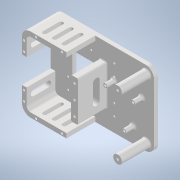
# Autodesk Inventor part: fleet
Saved by Autodesk Inventor 2020 (Build 240168000, 168)
## iProperties
Created: 2020-01-06
Part Number: fleet
Material: Generic
Document SubType Name: Modeling
Designer: my
Density: 1 g/cm^3
Appearance: Default
Author: my
Autodesk Inventor part; units mm, degrees
ref_plane "YZ Plane" through (0, 0, 0) normal (1, 0, 0) x (0, 1, 0)
ref_plane "XZ Plane" through (0, 0, 0) normal (0, 1, 0) x (-1, 0, 0)
ref_plane "XY Plane" through (0, 0, 0) normal (0, 0, 1) x (1, 0, 0)
sketch "Sketch1" plane through (0, 0, 0) normal (0, 0, 1) x (1, 0, 0)
  line L0 (-75, -65) -> (75, -65)
  line L1 (90, -50) -> (90, 50)
  line L2 (75, 65) -> (-75, 65)
  line L3 (-90, 50) -> (-90, -50)
  line L4 (-90, -65) -> (90, 65) construction
  line L5 (90, -65) -> (-90, 65) construction
  arc A0 (75, -65) -> (90, -50) centre (75, -50) ccw
  arc A1 (90, 50) -> (75, 65) centre (75, 50) ccw
  arc A2 (-75, 65) -> (-90, 50) centre (-75, 50) ccw
  arc A3 (-90, -50) -> (-75, -65) centre (-75, -50) ccw
  point P0 (0, 0)
  dimension "d0" = 180
  dimension "d1" = 130
  dimension "d9" = 15
  dimension "d10" = 15
  constraints: 12 end point, 8 point on circle, 8 point on line, 8 tangent, 4 centre point, 2 equal radius, 2 midpoint, 2 parallel, 1 horizontal, 1 perpendicular
  measures "d0" distance of L4.end L5.end
  measures "d1" distance of L5.start L4.end
  measures "d9" radius of A0
  measures "d10" radius of A1
extrude "Extrusion1" add sketch "Sketch1" along normal blind 7
sketch "Sketch3" plane through (0, 0, 7) normal (0, 0, 1) x (1, 0, 0)
  circle A0 centre (76.5, -52) radius 7.5
  circle A1 centre (76.5, 52) radius 7.5
  line L0 (7.5, 30) -> (-4.5, 30)
  line L1 (-4.5, 30) -> (-4.5, -30)
  line L2 (-4.5, -30) -> (7.5, -30)
  line L3 (7.5, -30) -> (7.5, 30)
  line L4 (7.5, 30) -> (-4.5, -30) construction
  line L5 (-4.5, 30) -> (7.5, -30) construction
  point P0 (1.5, 0)
  point P1 (0, 0)
  dimension "d11" = 15
  dimension "d12" = 104
  dimension "d13" = 52
  dimension "d14" = 75
  dimension "d15" = 12
  dimension "d16" = 60
  dimension "d17" = 7.5
  dimension "d18" = 30
  constraints: 12 end point, 2 centre point, 2 midpoint, 2 parallel, 1 equal radius, 1 horizontal, 1 perpendicular, 1 vertical alignment
  measures "d11" diameter of A0
  measures "d12" distance of A1.centre A0.centre
  measures "d13" vertical distance of point (1.5, 0) A0.centre
  measures "d14" horizontal distance of A0.centre point (1.5, 0)
  measures "d15" distance of L1.end L2.end
  measures "d16" distance of L0.end L1.end
  measures "d17" distance from line of point (0, 0) L3
  measures "d18" distance from line of L2 point (0, 0)
extrude "Extrusion2" add sketch "Sketch3" along normal blind 50
sketch "Sketch4" plane through (0, 0, 7) normal (0, 0, 1) x (1, 0, 0)
  line L0 (-12.5, 23) -> (-52.5, 23)
  line L1 (-52.5, 23) -> (-52.5, -23)
  line L2 (-52.5, -23) -> (-12.5, -23)
  line L3 (-12.5, -23) -> (-12.5, 23)
  line L4 (-12.5, 23) -> (-52.5, -23) construction
  line L5 (-52.5, 23) -> (-12.5, -23) construction
  line L6 (-4.5, -30) -> (-4.5, 30) projected
  point P0 (0, 0)
  point P1 (-32.5, 0)
  dimension "d21" = 46
  dimension "d22" = 40
  dimension "d25" = 28
  constraints: 12 end point, 2 midpoint, 2 parallel, 1 horizontal, 1 horizontal alignment, 1 perpendicular
  measures "d21" distance of L2.end L0.start
  measures "d22" distance of L1.end L2.end
  measures "d25" distance from line of L6 point (-32.5, 0)
extrude "Extrusion3" cut sketch "Sketch4" against normal mid plane 50
fillet "Fillet1" radius 2 8 edges at (1.5, 30, 7) (7.5, 0, 7) (7.5, 30, 32) (-4.5, 30, 32) (-4.5, 0, 7) (-4.5, -30, 32) (1.5, -30, 7) (7.5, -30, 32)
sketch "Sketch5" plane through (0, 0, 7) normal (0, 0, 1) x (1, 0, 0)
  arc A0 (90, 50) -> (75, 65) centre (75, 50) ccw projected
  line L0 (75, 65) -> (-75, 65) projected
  arc A1 (-75, 65) -> (-90, 50) centre (-75, 50) ccw projected
  line L1 (-90, 50) -> (-90, -50) projected
  arc A2 (-90, -50) -> (-75, -65) centre (-75, -50) ccw projected
  line L2 (-75, -65) -> (75, -65) projected
  arc A3 (75, -65) -> (90, -50) centre (75, -50) ccw projected
  line L3 (90, -50) -> (90, 50) projected
  circle A4 centre (76.5, -52) radius 7.5 projected
  circle A5 centre (76.5, 52) radius 7.5 projected
  line L4 (-52.5, 23) -> (-12.5, 23) projected
  line L5 (-12.5, 23) -> (-12.5, -23) projected
  line L6 (-12.5, -23) -> (-52.5, -23) projected
  line L7 (-52.5, -23) -> (-52.5, 23) projected
  arc A6 (-2.5, 32) -> (-6.5, 28) centre (-2.5, 28) ccw projected
  line L8 (5.5, 32) -> (-2.5, 32) projected
  arc A7 (9.5, 28) -> (5.5, 32) centre (5.5, 28) ccw projected
  line L9 (9.5, -28) -> (9.5, 28) projected
  arc A8 (5.5, -32) -> (9.5, -28) centre (5.5, -28) ccw projected
  line L10 (-2.5, -32) -> (5.5, -32) projected
  arc A9 (-6.5, -28) -> (-2.5, -32) centre (-2.5, -28) ccw projected
  line L11 (-6.5, 28) -> (-6.5, -28) projected
  line L12 (75, -57) -> (-75, -57)
  arc A10 (-82, -50) -> (-75, -57) centre (-75, -50) ccw
  line L13 (-82, -50) -> (-82, 50)
  arc A11 (-75, 57) -> (-82, 50) centre (-75, 50) ccw
  line L14 (-75, 57) -> (75, 57)
  arc A12 (82, 50) -> (75, 57) centre (75, 50) ccw
  line L15 (82, 50) -> (82, -50)
  arc A13 (75, -57) -> (82, -50) centre (75, -50) ccw
  line L16 (-82, -23) -> (-90, -23)
  line L17 (-82, 23) -> (-90, 23)
  line L18 (-12.5, -57) -> (-12.5, -65)
  line L19 (-12.5, 57) -> (-12.5, 65)
  line L20 (75, 65) -> (-75, 65) projected
  point P0 (0, 0)
  dimension "d27" = 8
  constraints: 16 end point, 14 point on line, 8 point on circle, 4 centre point, 1 collinear, 1 perpendicular, 7 other
  measures "d27" distance between parallel lines of L12 L2
extrude "Extrusion4" add sketch "Sketch5" along normal blind 50 contours L19 L14 A11 L13 L17 L1 A1 L0 | L2 A2 L1 L16 L13 A10 L12 L18
sketch "Sketch6" plane through (76.5, -52, 57) normal (0, 0, 1) x (1, 0, 0)
  circle A0 centre (0, 0) radius 7.5 projected
  circle A1 centre (0, 0) radius 2
  circle A2 centre (0, 104) radius 7.5 projected
  circle A3 centre (0, 104) radius 2
  circle A4 centre (-75, 27) radius 2
  circle A5 centre (-75, 52) radius 2
  circle A6 centre (-75, 77) radius 2
  circle A7 centre (-97, -9.5) radius 2
  circle A8 centre (-142, -9.5) radius 2
  circle A9 centre (-163, 6) radius 2
  circle A10 centre (-163, 23) radius 2
  circle A11 centre (-163, 81) radius 2
  circle A12 centre (-163, 98) radius 2
  circle A13 centre (-142, 113.5) radius 2
  circle A14 centre (-97, 113.5) radius 2
  line L0 (-81, 80) -> (-81, 24) projected
  line L1 (-151.5, -13) -> (-89, -13) projected
  line L2 (-89, -13) -> (-89, -5) projected
  line L3 (-166.5, 29) -> (-166.5, 2) projected
  line L4 (-158.5, 29) -> (-166.5, 29) projected
  line L5 (-166.5, 75) -> (-158.5, 75) projected
  line L6 (-166.5, 102) -> (-166.5, 75) projected
  line L7 (-89, 117) -> (-151.5, 117) projected
  point P0 (-76.5, 52)
  dimension "d30" = 4
  dimension "d31" = 6
  dimension "d32" = 25
  dimension "d33" = 25
  dimension "d34" = 45
  dimension "d35" = 3.5
  dimension "d36" = 8
  dimension "d37" = 3.5
  dimension "d38" = 17
  dimension "d39" = 6
  dimension "d40" = 6
  dimension "d41" = 3.5
  dimension "d42" = 17
  dimension "d43" = 3.5
  constraints: 13 centre point, 12 equal radius, 6 vertical alignment, 3 horizontal alignment, 2 coincident
  measures "d30" diameter of A1
  measures "d31" distance from line of A4.centre L0
  measures "d32" distance of A5.centre A4.centre
  measures "d33" distance of A6.centre A5.centre
  measures "d34" distance of A8.centre A7.centre
  measures "d35" distance from line of L1 A7.centre
  measures "d36" distance from line of A7.centre L2
  measures "d37" distance from line of L3 A9.centre
  measures "d38" distance of A10.centre A9.centre
  measures "d39" distance from line of L4 A10.centre
  measures "d40" distance from line of A11.centre L5
  measures "d41" distance from line of L6 A11.centre
  measures "d42" distance of A12.centre A11.centre
  measures "d43" distance from line of A14.centre L7
extrude "Extrusion5" cut sketch "Sketch6" against normal blind 10 contours A1 | A3 | A4 | A5 | A6 | A7 | A8 | A9 | A10 | A11 | A12 | A13 | A14
sketch "Sketch7" plane through (0, 0, 7) normal (0, 0, 1) x (1, 0, 0)
  point P0 (0, 0)
sketch "Sketch8" plane through (0, 0, 7) normal (0, 0, 1) x (1, 0, 0)
  circle A0 centre (20.7748, 40) radius 1.7 projected
  circle A1 centre (-59.5, 40) radius 1.7 projected
  circle A2 centre (-59.5, 20) radius 1.7 projected
  circle A3 centre (-19.3626, 40) radius 1.7 projected
  circle A4 centre (20.7748, 20) radius 1.7 projected
  arc A5 (-71.5, 50) -> (-74.5, 47) centre (-71.5, 47) ccw projected
  line L0 (-74.5, 0) -> (-74.5, 47) projected
  line L1 (-52.5, 0) -> (-74.5, 0) projected
  line L2 (-52.5, 23) -> (-52.5, 0) projected
  line L3 (-12.5, 23) -> (-52.5, 23) projected
  line L4 (-12.5, 0) -> (-12.5, 23) projected
  line L5 (-12.5, 0) -> (24.5, 0) projected
  line L6 (24.5, 47) -> (24.5, 0) projected
  arc A6 (24.5, 47) -> (21.5, 50) centre (21.5, 47) ccw projected
  line L7 (-71.5, 50) -> (21.5, 50) projected
  circle A7 centre (20.7748, -40) radius 1.7 projected
  circle A8 centre (-59.5, -40) radius 1.7 projected
  circle A9 centre (-59.5, -20) radius 1.7 projected
  circle A10 centre (-19.3626, -40) radius 1.7 projected
  circle A11 centre (20.7748, -20) radius 1.7 projected
  arc A12 (-74.5, -47) -> (-71.5, -50) centre (-71.5, -47) ccw projected
  line L8 (-71.5, -50) -> (21.5, -50) projected
  arc A13 (21.5, -50) -> (24.5, -47) centre (21.5, -47) ccw projected
  line L9 (24.5, -47) -> (24.5, 0) projected
  line L10 (-12.5, 0) -> (24.5, 0) projected
  line L11 (-12.5, 0) -> (-12.5, -23) projected
  line L12 (-12.5, -23) -> (-52.5, -23) projected
  line L13 (-52.5, -23) -> (-52.5, 0) projected
  line L14 (-52.5, 0) -> (-74.5, 0) projected
  line L15 (-74.5, 0) -> (-74.5, -47) projected
  point P0 (0, 0)
extrude "Extrusion6" cut sketch "Sketch8" against normal blind 10 contours A0 | A1 | A2 | A3 | A4 | A7 | A8 | A9 | A10 | A11
fillet "Fillet2" radius 2 2 edges at (69, 52, 7) (69, -52, 7)
sketch "Sketch10" plane through (0, 0, 7) normal (0, 0, 1) x (1, 0, 0)
  circle A0 centre (19.9935, 13.4034) radius 1.5875
  circle A1 centre (68.2535, 12.1314) radius 1.5875
  circle A2 centre (53.0135, -38.6666) radius 1.5875
  circle A3 centre (19.9935, 13.4034) radius 3.5
  circle A4 centre (68.2535, 12.1314) radius 3.5
  circle A5 centre (53.0135, -38.6666) radius 3.5
  point P0 (0, 0)
  dimension "d49" = 7
  constraints: 6 centre point, 3 coincident, 2 equal radius, 6 other
  measures "d49" diameter of A5
extrude "Extrusion7" add sketch "Sketch10" along normal blind 13 contours A0 | A1 | A2 | A3 | A4 | A5
fillet "Fillet3" radius 4 3 edges at (64.7535, 12.1314, 7) (16.4935, 13.4034, 7) (49.5135, -38.6666, 7)
sketch "Sketch11" plane through (19.9935, 13.4034, 20) normal (0, 0, 1) x (1, 0, 0)
  circle A0 centre (0, 0) radius 3.5 projected
  circle A1 centre (48.26, -1.272) radius 3.5 projected
  circle A2 centre (33.02, -52.07) radius 3.5 projected
  point P0 (-19.9935, -13.4034)
  constraints: 3 coincident
hole "Hole1" at (68.2535, 12.1314, 20) at (53.0135, -38.6666, 20) at (19.9935, 13.4034, 20) at (68.2535, 12.1314, 20) at (53.0135, -38.6666, 20) direction (0, 0, -1) diameter 4 depth 5 tip angle 118
sketch "Sketch12" plane through (-75, 65, 0) normal (0, 1, 0) x (1, 0, 0)
  line L0 (48, -18) -> (48, -46) construction
  line L1 (44.5, -18) -> (44.5, -46)
  line L2 (51.5, -46) -> (51.5, -18)
  arc A0 (51.5, -18) -> (44.5, -18) centre (48, -18) ccw
  arc A1 (44.5, -46) -> (51.5, -46) centre (48, -46) ccw
  line L3 (31, -18) -> (31, -46) construction
  line L4 (27.5, -18) -> (27.5, -46)
  line L5 (34.5, -46) -> (34.5, -18)
  arc A2 (34.5, -18) -> (27.5, -18) centre (31, -18) ccw
  arc A3 (27.5, -46) -> (34.5, -46) centre (31, -46) ccw
  line L6 (14, -18) -> (14, -46) construction
  line L7 (10.5, -18) -> (10.5, -46)
  line L8 (17.5, -46) -> (17.5, -18)
  arc A4 (17.5, -18) -> (10.5, -18) centre (14, -18) ccw
  arc A5 (10.5, -46) -> (17.5, -46) centre (14, -46) ccw
  line L9 (62.5, -57) -> (0, -57) projected
  line L10 (62.5, -7) -> (62.5, -57) projected
  point P0 (75, 0)
  point P1 (48, -32)
  point P2 (31, -32)
  point P3 (14, -32)
  dimension "d60" = 10
  dimension "d61" = 10
  dimension "d62" = 28
  dimension "d63" = 25
  dimension "d64" = 11
  dimension "d65" = 3.5
  constraints: 24 end point, 12 point on circle, 12 tangent, 6 centre point, 5 parallel, 3 midpoint, 3 vertical, 2 equal radius, 2 horizontal alignment
  measures "d60" distance between parallel lines of L4 L8
  measures "d61" distance between parallel lines of L1 L5
  measures "d62" distance of L5.start L5.end
  measures "d63" distance from line of L9 point (48, -32)
  measures "d64" distance between parallel lines of L10 L2
  measures "d65" radius of A0
extrude "Extrusion8" cut sketch "Sketch12" against normal through all
sketch "Sketch13" plane through (-4.5, -28, 57) normal (-1, 0, 0) x (0, 0, 1)
  line L0 (-32, 47) -> (-32, 17) construction
  line L1 (-38, 47) -> (-38, 17)
  line L2 (-26, 17) -> (-26, 47)
  arc A0 (-26, 47) -> (-38, 47) centre (-32, 47) ccw
  arc A1 (-38, 17) -> (-26, 17) centre (-32, 17) ccw
  line L3 (0, 0) -> (-48, 0) projected
  line L4 (-48, 0) -> (-48, 56) projected
  point P0 (-57, 28)
  point P1 (-32, 32)
  dimension "d68" = 30
  dimension "d69" = 12
  dimension "d70" = 32
  dimension "d71" = 16
  constraints: 8 end point, 4 point on circle, 4 tangent, 2 centre point, 1 midpoint, 1 parallel, 1 vertical
  measures "d68" distance of L1.start L1.end
  measures "d69" distance between parallel lines of L1 L2
  measures "d70" distance from line of L3 point (-32, 32)
  measures "d71" distance from line of L4 point (-32, 32)
extrude "Extrusion9" cut sketch "Sketch13" against normal blind 12
sketch "Sketch14" plane through (-90, -50, 0) normal (-1, 0, 0) x (0, 0, 1)
  line L0 (44.5, 87) -> (19.5, 87) construction
  line L1 (44.5, 92) -> (19.5, 92)
  line L2 (19.5, 82) -> (44.5, 82)
  arc A0 (44.5, 82) -> (44.5, 92) centre (44.5, 87) ccw
  arc A1 (19.5, 92) -> (19.5, 82) centre (19.5, 87) ccw
  line L3 (0, 100) -> (0, 0) projected
  line L4 (7, 73) -> (57, 73) projected
  line L5 (7, 27) -> (7, 73) projected
  line L6 (7, 50) -> (63.1063, 50) construction
  line L7 (44.5, 8) -> (19.5, 8)
  line L8 (19.5, 18) -> (44.5, 18)
  arc A2 (44.5, 8) -> (44.5, 18) centre (44.5, 13) ccw
  arc A3 (19.5, 18) -> (19.5, 8) centre (19.5, 13) ccw
  point P0 (0, 50)
  point P1 (32, 87)
  dimension "d74" = 25
  dimension "d75" = 5
  dimension "d76" = 32
  dimension "d77" = 14
  constraints: 14 end point, 8 point on circle, 6 symmetric about line, 4 centre point, 4 tangent, 2 horizontal, 2 midpoint, 1 parallel, 2 other
  measures "d74" distance of L0.start L0.end
  measures "d75" radius of A1
  measures "d76" distance from line of L3 point (32, 87)
  measures "d77" distance from line of L4 point (32, 87)
extrude "Extrusion10" cut sketch "Sketch14" against normal blind 12
body "Solid1"
